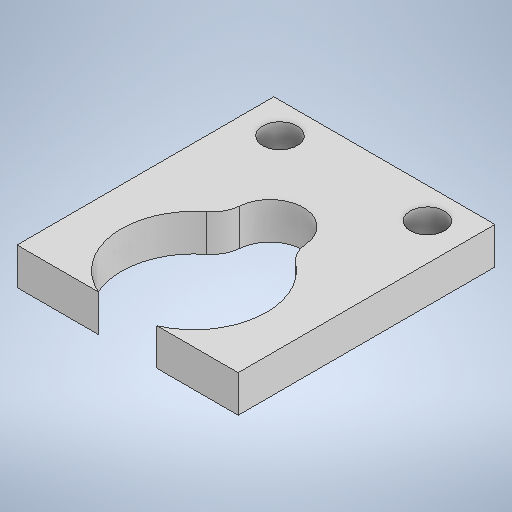
# Autodesk Inventor part: sujetador_cremallera
Saved by Autodesk Inventor 2025.2 (Build 292293000, 293)
## iProperties
Created: 2025-04-09
Part Number: sujetador_cremallera
Material: Generic
Document SubType Name: Modeling
Designer: cdavi
Density: 1 g/cm^3
Appearance: Default
Author: cdavi
Autodesk Inventor part; units mm, degrees
ref_plane "YZ Plane" through (0, 0, 0) normal (1, 0, 0) x (0, 1, 0)
ref_plane "XZ Plane" through (0, 0, 0) normal (0, 1, 0) x (-1, 0, 0)
ref_plane "XY Plane" through (0, 0, 0) normal (0, 0, 1) x (1, 0, 0)
sketch "Sketch2" plane through (0, 0, 0) normal (0, 1, 0) x (-1, 0, 0)
  circle A0 centre (0, 0) radius 2.7
  circle A1 centre (0, 6.2) radius 5.9
  line L0 (9, -9.3) -> (-9, -9.3)
  line L1 (-9, -9.3) -> (-9, 11.6)
  line L2 (-9, 11.6) -> (9, 11.6)
  line L3 (9, 11.6) -> (9, -9.3)
  circle A2 centre (6, -6.8) radius 1.4
  line L4 (0, 0) -> (0, -9.3) construction
  circle A3 centre (-6, -6.8) radius 1.4
  point P0 (2.377, 11.6)
  point P1 (2.5523, 0.8806)
  point P2 (-2.5523, 0.8806)
  point P3 (-2.377, 11.6)
  dimension "d20" = 5.4
  dimension "d21" = 11.8
  dimension "d22" = 6.2
  dimension "d23" = 5.4
  dimension "d24" = 18
  dimension "d25" = 20.9
  dimension "d26" = 2.8
  dimension "d27" = 2.5
  dimension "d28" = 3
  constraints: 10 end point, 4 centre point, 2 parallel, 2 perpendicular, 2 vertical alignment, 1 coincident, 1 horizontal, 1 midpoint, 1 symmetric about line, 1 other
  measures "d20" diameter of A0
  measures "d21" diameter of A1
  measures "d22" distance of A1.centre point (0, 0)
  measures "d23" distance from line of A1.centre L2
  measures "d24" distance of L0.start L0.end
  measures "d25" distance of L0.end L1.end
  measures "d26" diameter of A2
  measures "d27" distance from line of L0 A2.centre
  measures "d28" distance from line of L3 A2.centre
extrude "Extrusion1" add sketch "Sketch2" along normal blind 3 contours A0 A1 L2 L3 L0 L1
fillet "Fillet1" radius 2.5 2 edges at (-2.5523, 1.5, 0.8806) (2.5523, 1.5, 0.8806)
body "Solid1"
